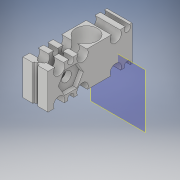
# Autodesk Inventor part: Neuroprobeholdermagiger for holding wires only
Saved by Autodesk Inventor 2017 (Build 210142000, 142)
## iProperties
Created: 2016-08-31
Part Number: Neuroprobeholdermagiger for holding wires only
Material: Generic
Document SubType Name: Modeling
Designer: andrew
Density: 1 g/cm^3
Appearance: Default
Author: andrew
Autodesk Inventor part; units mm, degrees
ref_plane "YZ Plane" through (0, 0, 0) normal (1, 0, 0) x (0, 1, 0)
ref_plane "XZ Plane" through (0, 0, 0) normal (0, 1, 0) x (-1, 0, 0)
ref_plane "XY Plane" through (0, 0, 0) normal (0, 0, 1) x (1, 0, 0)
sketch "Sketch1" plane through (0, 0, 0) normal (0, 1, 0) x (-1, 0, 0)
  line L0 (10.16, -5.2324) -> (10.16, -39.243)
  line L1 (0, -13.6734) -> (0, -5.2324)
  line L2 (0, -5.2324) -> (0, -39.243)
  line L3 (10.16, -39.243) -> (0, -39.243)
  arc A0 (4.064, -21.5807) -> (6.096, -21.5807) centre (5.08, -25.908) ccw
  line L4 (29.6544, -10.6206) -> (29.6544, -15.853) construction
  line L5 (29.6544, -10.6206) -> (34.8868, -10.6206) construction
  line L6 (4.064, -5.7752) -> (4.064, -5.2324)
  arc A1 (4.064, -7.1746) -> (4.064, -8.7525) centre (4.307, -7.9635) ccw
  line L7 (4.064, -7.1746) -> (4.064, -6.9486)
  line L8 (4.064, -5.2324) -> (4.064, -5.7752)
  line L9 (4.064, -6.9486) -> (4.064, -7.1746)
  arc A2 (6.0904, -8.7525) -> (6.0904, -7.1746) centre (5.8475, -7.9635) ccw
  line L10 (6.096, -5.7775) -> (6.096, -5.2324)
  line L11 (6.096, -5.2324) -> (6.096, -5.7775)
  line L12 (6.096, -6.9462) -> (6.096, -7.1763)
  line L13 (6.096, -7.1763) -> (6.096, -6.9462)
  line L14 (4.064, -8.7525) -> (4.064, -21.5807)
  line L15 (6.096, -21.5807) -> (6.096, -8.7507)
  line L16 (6.096, -5.2324) -> (10.16, -5.2324)
  line L17 (4.064, -5.2324) -> (0, -5.2324)
  arc A3 (6.096, -5.7775) -> (6.096, -6.9462) centre (5.8475, -6.3619) ccw
  arc A4 (4.064, -6.9486) -> (4.064, -5.7752) centre (4.307, -6.3619) ccw
  arc A5 (6.0904, -6.9486) -> (6.096, -6.9462) centre (5.8475, -6.3619) ccw
  arc A6 (6.096, -5.7775) -> (6.0904, -5.7752) centre (5.8475, -6.3619) ccw
  point P0 (0, 0)
  point P1 (6.096, -21.5807)
  dimension "d72" = 8.89
  dimension "d74" = 5.2324
  dimension "d75" = 90
  dimension "d112" = 10.16
  constraints: 36 end point, 18 point on circle, 7 centre point, 3 vertical, 2 perpendicular, 1 coincident, 1 horizontal, 1 parallel, 1 point on line
  measures "d72" diameter of A0
  measures "d74" distance of L4.start L4.end
  measures "d75" angle of L4 L5
  measures "d112" distance between parallel lines of L2 L0
extrude "Extrusion1" add sketch "Sketch1" along normal blind 19.05
sketch "Sketch2" plane through (0, 0, 0) normal (1, 0, 0) x (0, 0, -1)
  line L0 (20.9941, 0) -> (14.812, 0) construction
  line L1 (3.81, 19.05) -> (14.812, 19.05) construction
  line L2 (9.9978, 27.8595) -> (15.2302, 27.8595)
  line L3 (15.2302, 27.8595) -> (15.2302, 30.0439)
  line L4 (19.8791, 11.7094) -> (9.0424, 11.7094) construction
  circle A0 centre (14.4608, 11.7094) radius 1.8542
  point P0 (0, 0)
  point P1 (14.8101, 0)
  dimension "d77" = 5.2324
  dimension "d78" = 2.1844
  dimension "d79" = 3.7084
  constraints: 6 end point, 1 centre point, 1 horizontal, 1 midpoint, 1 perpendicular
  measures "d77" distance of L2.start L2.end
  measures "d78" distance of L2.end L3.end
  measures "d79" diameter of A0
extrude "Extrusion2" cut sketch "Sketch2" against normal blind 19.05
sketch "Sketch4" plane through (0, 0, 0) normal (1, 0, 0) x (0, 0, -1)
  line L0 (9.9598, 30.2256) -> (15.1922, 30.2256)
  line L1 (9.9598, 30.2256) -> (15.1922, 30.2256) construction
  line L2 (15.1922, 30.2256) -> (15.1922, 32.41)
  line L3 (19.5408, 11.7094) -> (17.0008, 7.31)
  line L4 (17.0008, 7.31) -> (11.9208, 7.31)
  line L5 (11.9208, 7.31) -> (9.3808, 11.7094)
  line L6 (9.3808, 11.7094) -> (11.9208, 16.1088)
  line L7 (11.9208, 16.1088) -> (17.0008, 16.1088)
  line L8 (17.0008, 16.1088) -> (19.5408, 11.7094)
  point P0 (0, 0)
  point P1 (9.2284, 9.525)
  point P2 (14.4608, 11.7094)
  dimension "d80" = 5.2324
  dimension "d81" = 0
  dimension "d82" = 2.1844
  dimension "d83" = 90
  dimension "d113" = 5.08
  constraints: 18 end point, 2 horizontal, 1 collinear, 1 perpendicular, 13 other
  measures "d80" distance of L0.start L0.end
  measures "d81" distance between parallel lines of L0 L1
  measures "d82" distance of L0.end L2.end
  measures "d83" angle of L2 L0
  measures "d113" distance of L6.end L7.end
extrude "Extrusion3" cut sketch "Sketch4" against normal blind 1.778
ref_plane "Work Plane1" through (0, 0, -33.528) normal (0, 0, -1) x (-1, 0, 0)
sketch "Sketch7" plane through (0, 0, 0) normal (1, 0, 0) x (0, 0, -1)
  line L0 (3.81, 19.05) -> (14.812, 19.05) projected
  line L1 (6.8407, 18.542) -> (6.8407, 19.05)
  line L2 (6.8407, 18.542) -> (7.3487, 18.542) construction
  line L3 (7.3243, 17.9943) -> (7.3243, 17.8356)
  line L4 (7.3243, 17.9943) -> (7.4831, 17.9943) construction
  circle A0 centre (19.1954, 17.5708) radius 2.286
  line L5 (5.2324, 0) -> (39.243, 0) projected
  line L6 (25.9172, 17.5708) -> (25.9172, -1.2171)
  line L7 (11.9208, 16.1088) -> (17.0008, 16.1088) projected
  line L8 (14.4608, 16.1088) -> (21.1986, 16.1088) construction
  circle A1 centre (14.4608, 18.0896) radius 1.27
  circle A2 centre (9.7261, 17.5708) radius 2.286
  line L9 (11.9208, 7.31) -> (9.3808, 11.7094) projected
  line L10 (9.3808, 11.7094) -> (19.5408, 11.7094)
  circle A3 centre (19.1954, 5.848) radius 2.286
  circle A4 centre (14.4608, 5.3292) radius 1.27
  circle A5 centre (9.7261, 5.848) radius 2.286
  circle A6 centre (32.639, 17.5708) radius 2.286
  circle A7 centre (37.3736, 18.0896) radius 1.27
  circle A8 centre (37.3736, 5.3292) radius 1.27
  circle A9 centre (32.639, 5.848) radius 2.286
  line L11 (-10.7191, 19.1949) -> (-10.7191, 18.6869)
  line L12 (-7.2754, 18.3631) -> (-7.2754, 18.6171)
  point P0 (0, 19.05)
  point P1 (30.353, 19.05)
  point P2 (30.353, 0)
  dimension "d42" = 0.508
  dimension "d43" = 90
  dimension "d46" = 0.1588
  dimension "d47" = 90
  dimension "d93" = 4.572
  dimension "d107" = 2.54
  dimension "d110" = 0.508
  dimension "d111" = 0.254
  constraints: 18 end point, 10 centre point, 4 horizontal, 3 vertical, 2 perpendicular, 1 midpoint
  measures "d42" distance of L1.start L1.end
  measures "d43" angle of L2 L1
  measures "d46" distance of L3.start L3.end
  measures "d47" angle of L3 L4
  measures "d93" diameter of A0
  measures "d107" diameter of A1
  measures "d110" distance of L11.start L11.end
  measures "d111" distance of L12.start L12.end
extrude "Extrusion6" cut sketch "Sketch7" against normal blind 55.88
sketch "Sketch9" plane through (-10.16, 0, -39.243) normal (-1, 0, 0) x (0, 0, 1)
  line L0 (36.3262, 29.806) -> (31.0938, 29.806)
  line L1 (31.0938, 29.806) -> (31.0938, 31.9904)
  circle A0 centre (24.7822, 11.7094) radius 2.0066
  point P0 (39.243, 0)
  dimension "d85" = 5.2324
  dimension "d86" = 2.1844
  dimension "d87" = 90
  dimension "d88" = 4.0132
  constraints: 4 end point, 1 centre point, 1 horizontal, 1 perpendicular
  measures "d85" distance of L0.start L0.end
  measures "d86" distance of L0.end L1.end
  measures "d87" angle of L0 L1
  measures "d88" diameter of A0
extrude "Extrusion8" cut sketch "Sketch9" against normal blind 12.7
fillet "Fillet2" radius 3.175 2 edges at (-6.096, 9.525, -21.5807) (-4.064, 9.525, -21.5807)
sketch "Sketch10" plane through (0, 0, -5.2324) normal (1, 0, 0) x (0, 0, -1)
  line L0 (11.7684, 7.31) -> (6.6884, 7.31) construction
  line L1 (6.6884, 7.31) -> (0, 7.31) construction
  line L2 (0, 7.31) -> (0, 4.77) construction
  line L3 (0, 4.77) -> (0, 4.77) construction
  line L4 (37.3327, 4.77) -> (37.3327, 5.086) construction
  line L5 (25.1206, 19.05) -> (25.1206, 0) construction
  line L6 (25.1206, 19.05) -> (27.6606, 19.05) construction
  line L7 (25.1206, 19.05) -> (27.6606, 19.05) construction
  line L8 (0, 0) -> (0, 19.05) construction
  line L9 (0, 4.77) -> (27.6606, 4.77) construction
  line L10 (39.4683, 4.77) -> (39.4683, -1.5422) construction
  line L11 (39.4683, -1.5422) -> (0, -1.5422) construction
  line L12 (0, -1.5422) -> (0, 4.77) construction
  line L13 (27.6606, 4.77) -> (0, 4.77) construction
  line L14 (39.4683, -1.5422) -> (0, -1.5422)
  line L15 (0, -1.5422) -> (0, 4.77)
  line L16 (0, 4.77) -> (27.6606, 4.77)
  line L17 (39.4683, -1.5422) -> (39.4683, 4.77)
  line L18 (27.6606, 4.77) -> (39.4683, 4.77)
  line L19 (39.4683, 22.6222) -> (39.4683, 19.05) construction
  line L20 (39.4683, 7.31) -> (39.4683, 4.77) construction
  point P0 (-5.2324, 0)
  dimension "d94" = 2.54
  dimension "d95" = 90
  dimension "d96" = 2.54
  dimension "d97" = 0
  constraints: 36 end point, 7 perpendicular, 5 horizontal, 4 point on line, 2 parallel, 1 collinear, 1 midpoint
  measures "d94" distance of L1.end L2.end
  measures "d95" angle of L3 L2
  measures "d96" distance of L6.start L6.end
  measures "d97" distance between parallel lines of L6 L7
extrude "Extrusion9" cut sketch "Sketch10" against normal blind 25.4
body "Solid1"
